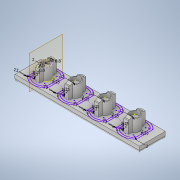
# Autodesk Inventor part: CapsFor24WellPlate
Saved by Autodesk Inventor 2021 (Build 250183000, 183)
## iProperties
Created: 2019-12-10
Part Number: CapsFor24WellPlate
Material: Generic
Document SubType Name: Modeling
Designer: Sergio
Density: 1 g/cm^3
Appearance: Default
Author: Sergio
Autodesk Inventor part; units mm, degrees
ref_plane "YZ Plane" through (0, 0, 0) normal (1, 0, 0) x (0, 1, 0)
ref_plane "XZ Plane" through (0, 0, 0) normal (0, 1, 0) x (-1, 0, 0)
ref_plane "XY Plane" through (0, 0, 0) normal (0, 0, 1) x (1, 0, 0)
sketch "Sketch1" plane through (0, 0, 0) normal (0, 1, 0) x (-1, 0, 0)
  circle A0 centre (-29.25, 0) radius 2.8 construction
  circle A1 centre (-9.75, 0) radius 2.8 construction
  circle A2 centre (9.75, 0) radius 2.8 construction
  circle A3 centre (29.25, 0) radius 2.8 construction
  line L0 (-29.25, 0) -> (29.25, 0) construction
  line L1 (29.25, 0) -> (29.25, -4.8) construction
  line L2 (9.75, 0) -> (9.75, -4.8) construction
  line L3 (-9.75, 0) -> (-9.75, -4.8) construction
  line L4 (-29.25, 0) -> (-29.25, -4.8) construction
  line L5 (29.25, 0) -> (29.25, 4.8) construction
  line L6 (9.75, 0) -> (9.75, 4.8) construction
  line L7 (-9.75, 0) -> (-9.75, 4.8) construction
  line L8 (-29.25, 0) -> (-29.25, 4.8) construction
  line L9 (30.65, -5.6) -> (27.85, -5.6) construction
  line L10 (27.85, -5.6) -> (27.85, -4.8) construction
  line L11 (27.85, -4.8) -> (30.65, -4.8) construction
  line L12 (30.65, -4.8) -> (30.65, -5.6) construction
  line L13 (11.15, -5.6) -> (8.35, -5.6) construction
  line L14 (8.35, -5.6) -> (8.35, -4.8) construction
  line L15 (8.35, -4.8) -> (11.15, -4.8) construction
  line L16 (11.15, -4.8) -> (11.15, -5.6) construction
  line L17 (-8.35, -5.6) -> (-11.15, -5.6) construction
  line L18 (-11.15, -5.6) -> (-11.15, -4.8) construction
  line L19 (-11.15, -4.8) -> (-8.35, -4.8) construction
  line L20 (-8.35, -4.8) -> (-8.35, -5.6) construction
  line L21 (-27.85, -5.6) -> (-30.65, -5.6) construction
  line L22 (-30.65, -5.6) -> (-30.65, -4.8) construction
  line L23 (-30.65, -4.8) -> (-27.85, -4.8) construction
  line L24 (-27.85, -4.8) -> (-27.85, -5.6) construction
  line L25 (27.85, 5.6) -> (30.65, 5.6) construction
  line L26 (30.65, 5.6) -> (30.65, 4.8) construction
  line L27 (30.65, 4.8) -> (27.85, 4.8) construction
  line L28 (27.85, 4.8) -> (27.85, 5.6) construction
  line L29 (8.35, 5.6) -> (11.15, 5.6) construction
  line L30 (11.15, 5.6) -> (11.15, 4.8) construction
  line L31 (11.15, 4.8) -> (8.35, 4.8) construction
  line L32 (8.35, 4.8) -> (8.35, 5.6) construction
  line L33 (-11.15, 5.6) -> (-8.35, 5.6) construction
  line L34 (-8.35, 5.6) -> (-8.35, 4.8) construction
  line L35 (-8.35, 4.8) -> (-11.15, 4.8) construction
  line L36 (-11.15, 4.8) -> (-11.15, 5.6) construction
  line L37 (-30.65, 5.6) -> (-27.85, 5.6) construction
  line L38 (-27.85, 5.6) -> (-27.85, 4.8) construction
  line L39 (-27.85, 4.8) -> (-30.65, 4.8) construction
  line L40 (-30.65, 4.8) -> (-30.65, 5.6) construction
  dimension "d171" = 2.8
  dimension "d172" = 0.8
  dimension "d173" = 2.8
  dimension "d174" = 0.8
  dimension "d175" = 2.8
  dimension "d176" = 0.8
  dimension "d177" = 2.8
  dimension "d178" = 0.8
  dimension "d179" = 2.8
  dimension "d180" = 0.8
  dimension "d181" = 2.8
  dimension "d182" = 0.8
  dimension "d183" = 2.8
  dimension "d184" = 0.8
  dimension "d185" = 2.8
  dimension "d186" = 0.8
  constraints: 82 end point, 16 parallel, 8 midpoint, 8 perpendicular, 5 horizontal, 4 centre point, 4 vertical
  measures "d171" distance of L10.end L11.end
  measures "d172" distance of L10.start L10.end
  measures "d173" distance of L14.end L15.end
  measures "d174" distance of L14.start L14.end
  measures "d175" distance of L18.end L19.end
  measures "d176" distance of L18.start L18.end
  measures "d177" distance of L22.end L23.end
  measures "d178" distance of L22.start L22.end
  measures "d179" distance of L27.start L28.start
  measures "d180" distance of L25.end L27.start
  measures "d181" distance of L31.start L32.start
  measures "d182" distance of L29.end L31.start
  measures "d183" distance of L35.start L36.start
  measures "d184" distance of L33.end L35.start
  measures "d185" distance of L39.start L40.start
  measures "d186" distance of L37.end L39.start
sketch "Sketch26" plane through (0, 0, 0) normal (0, 1, 0) x (-1, 0, 0)
  line L0 (-41, -8.5) -> (41, -8.5)
  line L1 (41, -8.5) -> (41, 8.5)
  line L2 (41, 8.5) -> (-41, 8.5)
  line L3 (-41, 8.5) -> (-41, -8.5)
  line L4 (-41, -8.5) -> (41, 8.5) construction
  line L5 (41, -8.5) -> (-41, 8.5) construction
  point P0 (0, 0)
  dimension "d187" = 82
  dimension "d188" = 17
  constraints: 12 end point, 2 midpoint, 2 parallel, 1 horizontal, 1 perpendicular
  measures "d187" distance of L2.end L1.end
  measures "d188" distance of L1.end L0.end
extrude "Extrusion11" add sketch "Sketch26" against normal blind 4.5
sketch "Sketch27" plane through (0, 0, 0) normal (0, 1, 0) x (1, 0, 0)
  circle A0 centre (-29.25, 0) radius 2.8 construction
  circle A1 centre (-9.75, 0) radius 2.8 construction
  circle A2 centre (9.75, 0) radius 2.8 construction
  circle A3 centre (29.25, 0) radius 2.8 construction
  line L0 (-30.65, 5.6) -> (-27.85, 5.6) construction
  line L1 (-27.85, 4.8) -> (-30.65, 4.8) construction
  line L2 (-11.15, 5.6) -> (-8.35, 5.6) construction
  line L3 (-8.35, 4.8) -> (-11.15, 4.8) construction
  line L4 (8.35, 5.6) -> (11.15, 5.6) construction
  line L5 (11.15, 4.8) -> (8.35, 4.8) construction
  line L6 (30.65, 4.8) -> (27.85, 4.8) construction
  line L7 (27.85, 5.6) -> (30.65, 5.6) construction
  line L8 (-27.85, -5.6) -> (-30.65, -5.6) construction
  line L9 (-30.65, -4.8) -> (-27.85, -4.8) construction
  circle A4 centre (-29.25, 0) radius 3.325
  circle A5 centre (-9.75, 0) radius 3.325
  circle A6 centre (9.75, 0) radius 3.325
  circle A7 centre (29.25, 0) radius 3.325
  line L10 (-11.15, 5.6) -> (-8.35, 5.6)
  line L11 (-8.35, 5.6) -> (-8.35, 4.8)
  line L12 (-8.35, 4.8) -> (-11.15, 4.8)
  line L13 (-11.15, 4.8) -> (-11.15, 5.6)
  line L14 (8.35, 5.6) -> (11.15, 5.6)
  line L15 (11.15, 5.6) -> (11.15, 4.8)
  line L16 (11.15, 4.8) -> (8.35, 4.8)
  line L17 (8.35, 4.8) -> (8.35, 5.6)
  line L18 (27.85, 5.6) -> (30.65, 5.6)
  line L19 (30.65, 5.6) -> (30.65, 4.8)
  line L20 (30.65, 4.8) -> (27.85, 4.8)
  line L21 (27.85, 4.8) -> (27.85, 5.6)
  line L22 (-30.65, 5.6) -> (-27.85, 5.6)
  line L23 (-27.85, 5.6) -> (-27.85, 4.8)
  line L24 (-27.85, 4.8) -> (-30.65, 4.8)
  line L25 (-30.65, 4.8) -> (-30.65, 5.6)
  line L26 (-30.65, -4.8) -> (-27.85, -4.8)
  line L27 (-27.85, -4.8) -> (-27.85, -5.6)
  line L28 (-27.85, -5.6) -> (-30.65, -5.6)
  line L29 (-30.65, -5.6) -> (-30.65, -4.8)
  line L30 (-8.35, -5.6) -> (-11.15, -5.6) construction
  line L31 (-11.15, -4.8) -> (-8.35, -4.8) construction
  line L32 (11.15, -5.6) -> (8.35, -5.6) construction
  line L33 (8.35, -4.8) -> (11.15, -4.8) construction
  line L34 (30.65, -5.6) -> (27.85, -5.6) construction
  line L35 (27.85, -4.8) -> (30.65, -4.8) construction
  line L36 (-11.15, -4.8) -> (-8.35, -4.8)
  line L37 (-8.35, -4.8) -> (-8.35, -5.6)
  line L38 (-8.35, -5.6) -> (-11.15, -5.6)
  line L39 (-11.15, -5.6) -> (-11.15, -4.8)
  line L40 (8.35, -4.8) -> (11.15, -4.8)
  line L41 (11.15, -4.8) -> (11.15, -5.6)
  line L42 (11.15, -5.6) -> (8.35, -5.6)
  line L43 (8.35, -5.6) -> (8.35, -4.8)
  line L44 (27.85, -4.8) -> (30.65, -4.8)
  line L45 (30.65, -4.8) -> (30.65, -5.6)
  line L46 (30.65, -5.6) -> (27.85, -5.6)
  line L47 (27.85, -5.6) -> (27.85, -4.8)
  line L48 (-30.65, 4.8) -> (-30.65, -4.8)
  line L49 (-27.85, 4.8) -> (-27.85, -4.8)
  line L50 (-11.15, 4.8) -> (-11.15, -4.8)
  line L51 (-8.35, 4.8) -> (-8.35, -4.8)
  line L52 (27.85, 4.8) -> (27.85, -4.8)
  line L53 (30.65, -4.8) -> (30.65, 4.8)
  line L54 (8.35, 4.8) -> (8.35, -4.8)
  line L55 (11.15, -4.8) -> (11.15, 4.8)
  point P0 (0, 0)
  dimension "d191" = 6.65
  dimension "d192" = 6.65
  dimension "d193" = 6.65
  dimension "d194" = 6.65
  constraints: 80 end point, 22 parallel, 10 perpendicular, 8 horizontal, 4 centre point, 4 coincident
  measures "d191" diameter of A4
  measures "d192" diameter of A5
  measures "d193" diameter of A6
  measures "d194" diameter of A7
extrude "Extrusion12" add sketch "Sketch27" along normal blind 8
sketch "Sketch28" plane through (0, 8, 0) normal (0, 1, 0) x (1, 0, 0)
  arc A0 (-30.65, 3.0159) -> (-30.65, -3.0159) centre (-29.25, 0) ccw projected
  circle A1 centre (-29.25, 0) radius 2.825
  arc A2 (-8.35, -3.0159) -> (-8.35, 3.0159) centre (-9.75, 0) ccw projected
  circle A3 centre (-9.75, 0) radius 2.825
  arc A4 (11.15, -3.0159) -> (11.15, 3.0159) centre (9.75, 0) ccw projected
  circle A5 centre (9.75, 0) radius 2.825
  arc A6 (30.65, -3.0159) -> (30.65, 3.0159) centre (29.25, 0) ccw projected
  circle A7 centre (29.25, 0) radius 2.825
  point P0 (0, 0)
  dimension "d197" = 5.65
  dimension "d198" = 5.65
  dimension "d199" = 5.65
  dimension "d200" = 5.65
  constraints: 4 centre point, 4 coincident
  measures "d197" diameter of A1
  measures "d198" diameter of A3
  measures "d199" diameter of A5
  measures "d200" diameter of A7
extrude "Extrusion13" cut sketch "Sketch28" against normal blind 2
sketch "Sketch29" plane through (0, 8, 0) normal (0, 1, 0) x (1, 0, 0)
  line L0 (-27.85, 5.6) -> (-30.65, 5.6) construction
  line L1 (-30.65, 5.6) -> (-27.85, 5.6) construction
  line L2 (-27.85, 5.6) -> (-27.85, 4.8) construction
  line L3 (-27.85, 4.8) -> (-30.65, 4.8) construction
  line L4 (-30.65, 4.8) -> (-30.65, 5.6) construction
  line L5 (-30.65, -3.0159) -> (-30.65, -5.6) construction
  line L6 (-30.65, -5.6) -> (-27.85, -5.6) construction
  line L7 (-27.85, -5.6) -> (-27.85, -4.8) construction
  line L8 (-27.85, -4.8) -> (-30.65, -4.8) construction
  line L9 (-30.65, -4.8) -> (-30.65, -5.6) construction
  arc A0 (-27.85, -3.0159) -> (-27.85, 3.0159) centre (-29.25, 0) ccw construction
  circle A1 centre (-29.25, 0) radius 3.325 construction
  line L10 (-29.25, 0) -> (-26.425, 0) construction
  circle A2 centre (-29.25, 0) radius 2.825 construction
  point P0 (-9.75, 0)
  point P1 (9.75, 0)
  point P2 (29.25, 0)
  dimension "d203" = 2.8
  dimension "d204" = 0.8
  dimension "d205" = 2.8
  dimension "d206" = 0.8
  constraints: 18 end point, 4 parallel, 3 horizontal, 2 coincident, 2 perpendicular, 1 centre point, 1 horizontal alignment, 1 other
  measures "d203" distance of L2.end L3.end
  measures "d204" distance of L1.end L2.end
  measures "d205" distance of L8.end L7.end
  measures "d206" distance of L7.end L6.end
ref_plane "Work Plane7" through (-29.25, 8, 0) normal (1, 0, 0) x (0, 1, 0)
sketch "Sketch30" plane through (-29.25, 8, 0) normal (1, 0, 0) x (0, 1, 0)
  line L0 (0, -3.325) -> (0, 3.325) construction
  line L1 (0, 4.8) -> (0, 3.325)
  line L2 (0, 3.325) -> (1, 3.325)
  line L3 (1, 3.325) -> (0, 4.8)
  line L4 (0, -4.8) -> (0, -3.325)
  line L5 (0, -3.325) -> (1, -3.325)
  line L6 (1, -3.325) -> (0, -4.8)
  point P0 (-8, 0)
  dimension "d207" = 1
  dimension "d210" = 1
  constraints: 12 end point, 2 vertical, 1 horizontal, 1 perpendicular
  measures "d207" distance of L0.end L2.end
  measures "d210" distance of L0.start L5.end
extrude "Extrusion14" add sketch "Sketch30" along normal mid plane 2.8 contours L3 L2 L1
extrude "Extrusion15" add sketch "Sketch30" along normal mid plane 2.8 contours L4 L5 L6
sketch "Sketch31" plane through (0, 8, 0) normal (0, 1, 0) x (1, 0, 0)
  line L0 (-30.65, -3.325) -> (-27.85, -3.325) projected
  arc A0 (-27.85, -3.0159) -> (-27.85, 3.0159) centre (-29.25, 0) ccw projected
  line L1 (-27.85, -3.325) -> (-27.85, -3.0159) projected
  line L2 (-27.85, -3.325) -> (-27.85, -3.0159)
  line L3 (-27.85, -3.325) -> (-29.25, -3.325)
  line L4 (-30.65, -3.0159) -> (-30.65, -3.325) projected
  arc A1 (-30.65, 3.0159) -> (-30.65, -3.0159) centre (-29.25, 0) ccw projected
  line L5 (-30.65, -3.0159) -> (-30.65, -3.325)
  line L6 (-30.65, -3.325) -> (-29.25, -3.325)
  line L7 (-27.85, 3.325) -> (-30.65, 3.325) projected
  line L8 (-30.65, 3.0159) -> (-30.65, 3.325)
  line L9 (-27.85, 3.0159) -> (-27.85, 3.325)
  line L10 (-27.85, 3.325) -> (-29.25, 3.325)
  line L11 (-29.25, 3.325) -> (-30.65, 3.325)
  line L12 (-30.65, -3.0159) -> (-30.65, -2.4537)
  circle A2 centre (-29.25, 0) radius 2.825 projected
  line L13 (-27.85, -3.0159) -> (-27.85, -2.4537)
  arc A3 (-30.65, -2.4537) -> (-27.85, -2.4537) centre (-29.25, 0) ccw
  line L14 (-30.65, 3.0159) -> (-30.65, 2.4537)
  line L15 (-27.85, 3.0159) -> (-27.85, 2.4537)
  arc A4 (-27.85, 2.4537) -> (-30.65, 2.4537) centre (-29.25, 0) ccw
  point P0 (0, 0)
  constraints: 24 end point, 8 point on circle, 3 collinear, 3 perpendicular, 3 vertical, 2 centre point, 2 concentric, 2 midpoint, 1 parallel, 1 point on line
fillet "Fillet2" radius 2 4 edges at (0, -4.5, -8.5) (0, -4.5, 8.5) (41, -4.5, 0) (-41, -4.5, 0)
sketch "Sketch33" plane through (0, 8, 0) normal (0, 1, 0) x (1, 0, 0)
  circle A0 centre (-9.75, 0) radius 2.825 projected
  circle A1 centre (9.75, 0) radius 2.825 projected
  circle A2 centre (29.25, 0) radius 2.825 projected
  point P0 (0, 0)
  constraints: 3 coincident
extrude "Extrusion19" add sketch "Sketch31" along normal blind 1 contours L4 L12 A2 L13 L1 L0 | L8 L7 L9 L15 A2 L14
pattern_sketch "Sketch Driven Pattern3" of "Extrusion14", "Extrusion19", "Extrusion15" from (-29.25, 8, 0) copies at (-9.75, 8, 0) at (9.75, 8, 0) at (29.25, 8, 0)
sketch "Sketch34" plane through (0, 0, 0) normal (0, 1, 0) x (1, 0, 0)
  circle A0 centre (-29.25, 0) radius 2.8 construction
  line L0 (-22, 0) -> (-26.45, 0) construction
  arc A1 (-30.65, 3.0159) -> (-30.65, -3.0159) centre (-29.25, 0) ccw projected
  line L1 (-32.575, 0) -> (-34.575, 0) construction
  line L2 (-34.575, 0) -> (-34.575, 4.0629)
  line L3 (-34.575, 0) -> (-34.575, -4.0629)
  line L4 (-34.575, 0) -> (-35.825, 0) construction
  line L5 (-35.825, 0) -> (-35.825, 4.6173)
  line L6 (-35.825, 0) -> (-35.825, -4.6173)
  arc A2 (-35.825, -4.6173) -> (-35.2327, -6.038) centre (-33.825, -4.6173) ccw
  arc A3 (-34.575, -4.0629) -> (-33.8417, -5.6106) centre (-32.575, -4.0629) ccw
  arc A4 (-33.8417, 5.6106) -> (-34.575, 4.0629) centre (-32.575, 4.0629) ccw
  arc A5 (-35.2327, 6.038) -> (-35.825, 4.6173) centre (-33.825, 4.6173) ccw
  arc A6 (-27.85, -3.0159) -> (-27.85, 3.0159) centre (-29.25, 0) ccw projected
  line L7 (-25.925, 0) -> (-23.925, 0) construction
  line L8 (-23.925, 0) -> (-22.675, 0) construction
  line L9 (-23.925, 0) -> (-23.925, 4.0629)
  line L10 (-23.925, 0) -> (-23.925, -4.0629)
  line L11 (-22.675, 0) -> (-22.675, 4.6173)
  line L12 (-22.675, 0) -> (-22.675, -4.6173)
  arc A7 (-35.2327, -6.038) -> (-23.2673, -6.038) centre (-29.25, 0) ccw
  arc A8 (-23.2673, 6.038) -> (-35.2327, 6.038) centre (-29.25, 0) ccw
  arc A9 (-33.8417, -5.6106) -> (-24.6583, -5.6106) centre (-29.25, 0) ccw
  arc A10 (-24.6583, 5.6106) -> (-33.8417, 5.6106) centre (-29.25, 0) ccw
  arc A11 (-24.6583, -5.6106) -> (-23.925, -4.0629) centre (-25.925, -4.0629) ccw
  arc A12 (-23.2673, -6.038) -> (-22.675, -4.6173) centre (-24.675, -4.6173) ccw
  arc A13 (-22.675, 4.6173) -> (-23.2673, 6.038) centre (-24.675, 4.6173) ccw
  arc A14 (-23.925, 4.0629) -> (-24.6583, 5.6106) centre (-25.925, 4.0629) ccw
  circle A15 centre (-32.575, -4.0629) radius 1
  circle A16 centre (-9.75, 0) radius 2.825 projected
  circle A17 centre (9.75, 0) radius 2.825 projected
  circle A18 centre (29.25, 0) radius 2.825 projected
  line L13 (-2.5, 0) -> (-6.95, 0) construction
  line L14 (-13.075, 0) -> (-15.075, 0) construction
  line L15 (-15.075, 0) -> (-15.075, 4.0629)
  line L16 (-15.075, 0) -> (-15.075, -4.0629)
  line L17 (-15.075, 0) -> (-16.325, 0) construction
  line L18 (-16.325, 0) -> (-16.325, 4.6173)
  line L19 (-16.325, 0) -> (-16.325, -4.6173)
  arc A19 (-16.325, -4.6173) -> (-15.7327, -6.038) centre (-14.325, -4.6173) ccw
  arc A20 (-15.075, -4.0629) -> (-14.3417, -5.6106) centre (-13.075, -4.0629) ccw
  arc A21 (-14.3417, 5.6106) -> (-15.075, 4.0629) centre (-13.075, 4.0629) ccw
  arc A22 (-15.7327, 6.038) -> (-16.325, 4.6173) centre (-14.325, 4.6173) ccw
  line L20 (-6.425, 0) -> (-4.425, 0) construction
  line L21 (-4.425, 0) -> (-3.175, 0) construction
  line L22 (-4.425, 0) -> (-4.425, 4.0629)
  line L23 (-4.425, 0) -> (-4.425, -4.0629)
  line L24 (-3.175, 0) -> (-3.175, 4.6173)
  line L25 (-3.175, 0) -> (-3.175, -4.6173)
  arc A23 (-15.7327, -6.038) -> (-3.7673, -6.038) centre (-9.75, 0) ccw
  arc A24 (-3.7673, 6.038) -> (-15.7327, 6.038) centre (-9.75, 0) ccw
  arc A25 (-14.3417, -5.6106) -> (-5.1583, -5.6106) centre (-9.75, 0) ccw
  arc A26 (-5.1583, 5.6106) -> (-14.3417, 5.6106) centre (-9.75, 0) ccw
  arc A27 (-5.1583, -5.6106) -> (-4.425, -4.0629) centre (-6.425, -4.0629) ccw
  arc A28 (-3.7673, -6.038) -> (-3.175, -4.6173) centre (-5.175, -4.6173) ccw
  arc A29 (-3.175, 4.6173) -> (-3.7673, 6.038) centre (-5.175, 4.6173) ccw
  arc A30 (-4.425, 4.0629) -> (-5.1583, 5.6106) centre (-6.425, 4.0629) ccw
  circle A31 centre (-13.075, -4.0629) radius 1
  line L26 (17, 0) -> (12.55, 0) construction
  line L27 (6.425, 0) -> (4.425, 0) construction
  line L28 (4.425, 0) -> (4.425, 4.0629)
  line L29 (4.425, 0) -> (4.425, -4.0629)
  line L30 (4.425, 0) -> (3.175, 0) construction
  line L31 (3.175, 0) -> (3.175, 4.6173)
  line L32 (3.175, 0) -> (3.175, -4.6173)
  arc A32 (3.175, -4.6173) -> (3.7673, -6.038) centre (5.175, -4.6173) ccw
  arc A33 (4.425, -4.0629) -> (5.1583, -5.6106) centre (6.425, -4.0629) ccw
  arc A34 (5.1583, 5.6106) -> (4.425, 4.0629) centre (6.425, 4.0629) ccw
  arc A35 (3.7673, 6.038) -> (3.175, 4.6173) centre (5.175, 4.6173) ccw
  line L33 (13.075, 0) -> (15.075, 0) construction
  line L34 (15.075, 0) -> (16.325, 0) construction
  line L35 (15.075, 0) -> (15.075, 4.0629)
  line L36 (15.075, 0) -> (15.075, -4.0629)
  line L37 (16.325, 0) -> (16.325, 4.6173)
  line L38 (16.325, 0) -> (16.325, -4.6173)
  arc A36 (3.7673, -6.038) -> (15.7327, -6.038) centre (9.75, 0) ccw
  arc A37 (15.7327, 6.038) -> (3.7673, 6.038) centre (9.75, 0) ccw
  arc A38 (5.1583, -5.6106) -> (14.3417, -5.6106) centre (9.75, 0) ccw
  arc A39 (14.3417, 5.6106) -> (5.1583, 5.6106) centre (9.75, 0) ccw
  arc A40 (14.3417, -5.6106) -> (15.075, -4.0629) centre (13.075, -4.0629) ccw
  arc A41 (15.7327, -6.038) -> (16.325, -4.6173) centre (14.325, -4.6173) ccw
  arc A42 (16.325, 4.6173) -> (15.7327, 6.038) centre (14.325, 4.6173) ccw
  arc A43 (15.075, 4.0629) -> (14.3417, 5.6106) centre (13.075, 4.0629) ccw
  circle A44 centre (6.425, -4.0629) radius 1
  line L39 (36.5, 0) -> (32.05, 0) construction
  line L40 (25.925, 0) -> (23.925, 0) construction
  line L41 (23.925, 0) -> (23.925, 4.0629)
  line L42 (23.925, 0) -> (23.925, -4.0629)
  line L43 (23.925, 0) -> (22.675, 0) construction
  line L44 (22.675, 0) -> (22.675, 4.6173)
  line L45 (22.675, 0) -> (22.675, -4.6173)
  arc A45 (22.675, -4.6173) -> (23.2673, -6.038) centre (24.675, -4.6173) ccw
  arc A46 (23.925, -4.0629) -> (24.6583, -5.6106) centre (25.925, -4.0629) ccw
  arc A47 (24.6583, 5.6106) -> (23.925, 4.0629) centre (25.925, 4.0629) ccw
  arc A48 (23.2673, 6.038) -> (22.675, 4.6173) centre (24.675, 4.6173) ccw
  line L46 (32.575, 0) -> (34.575, 0) construction
  line L47 (34.575, 0) -> (35.825, 0) construction
  line L48 (34.575, 0) -> (34.575, 4.0629)
  line L49 (34.575, 0) -> (34.575, -4.0629)
  line L50 (35.825, 0) -> (35.825, 4.6173)
  line L51 (35.825, 0) -> (35.825, -4.6173)
  arc A49 (23.2673, -6.038) -> (35.2327, -6.038) centre (29.25, 0) ccw
  arc A50 (35.2327, 6.038) -> (23.2673, 6.038) centre (29.25, 0) ccw
  arc A51 (24.6583, -5.6106) -> (33.8417, -5.6106) centre (29.25, 0) ccw
  arc A52 (33.8417, 5.6106) -> (24.6583, 5.6106) centre (29.25, 0) ccw
  arc A53 (33.8417, -5.6106) -> (34.575, -4.0629) centre (32.575, -4.0629) ccw
  arc A54 (35.2327, -6.038) -> (35.825, -4.6173) centre (33.825, -4.6173) ccw
  arc A55 (35.825, 4.6173) -> (35.2327, 6.038) centre (33.825, 4.6173) ccw
  arc A56 (34.575, 4.0629) -> (33.8417, 5.6106) centre (32.575, 4.0629) ccw
  circle A57 centre (25.925, -4.0629) radius 1
  point P0 (-35.825, 5.387)
  point P1 (-35.825, -5.387)
  point P2 (-34.575, 4.92)
  point P3 (-34.575, -4.92)
  point P4 (-22.675, 5.387)
  point P5 (-22.675, -5.387)
  point P6 (-23.925, 4.92)
  point P7 (-23.925, -4.92)
  point P8 (-16.325, 5.387)
  point P9 (-16.325, -5.387)
  point P10 (-15.075, 4.92)
  point P11 (-15.075, -4.92)
  point P12 (-3.175, 5.387)
  point P13 (-3.175, -5.387)
  point P14 (-4.425, 4.92)
  point P15 (-4.425, -4.92)
  point P16 (3.175, 5.387)
  point P17 (3.175, -5.387)
  point P18 (4.425, 4.92)
  point P19 (4.425, -4.92)
  point P20 (16.325, 5.387)
  point P21 (16.325, -5.387)
  point P22 (15.075, 4.92)
  point P23 (15.075, -4.92)
  point P24 (22.675, 5.387)
  point P25 (22.675, -5.387)
  point P26 (23.925, 4.92)
  point P27 (23.925, -4.92)
  point P28 (35.825, 5.387)
  point P29 (35.825, -5.387)
  point P30 (34.575, 4.92)
  point P31 (34.575, -4.92)
  dimension "d242" = 2
  dimension "d243" = 1.25
  dimension "d244" = 2
  dimension "d245" = 2
  dimension "d246" = 2
  dimension "d247" = 2
  dimension "d248" = 1.25
  dimension "d249" = 2
  dimension "d250" = 2
  dimension "d251" = 2
  dimension "d252" = 1.25
  dimension "d253" = 2
  dimension "d254" = 2
  dimension "d255" = 2
  dimension "d256" = 2
  dimension "d257" = 1.25
  dimension "d258" = 2
  dimension "d259" = 2
  dimension "d260" = 2
  dimension "d261" = 1.25
  dimension "d262" = 2
  dimension "d263" = 2
  dimension "d264" = 2
  dimension "d265" = 2
  dimension "d266" = 1.25
  dimension "d267" = 2
  dimension "d268" = 2
  dimension "d269" = 2
  dimension "d270" = 1.25
  dimension "d271" = 2
  dimension "d272" = 2
  dimension "d273" = 2
  dimension "d274" = 2
  dimension "d275" = 1.25
  dimension "d276" = 2
  dimension "d277" = 2
  constraints: 114 point on circle, 104 end point, 52 centre point, 48 point on line, 48 tangent, 24 vertical, 16 equal radius, 12 coincident, 8 horizontal, 1 horizontal alignment, 1 other
  measures "d242" distance of L1.start L1.end
  measures "d243" distance of L1.end L4.end
  measures "d244" radius of A2
  measures "d245" radius of A3
  measures "d246" radius of A4
  measures "d247" distance of L7.start L7.end
  measures "d248" distance of L7.end L8.end
  measures "d249" radius of A11
  measures "d250" diameter of A15
  measures "d251" distance of L14.start L14.end
  measures "d252" distance of L14.end L17.end
  measures "d253" radius of A19
  measures "d254" radius of A20
  measures "d255" radius of A21
  measures "d256" distance of L20.start L20.end
  measures "d257" distance of L20.end L24.start
  measures "d258" radius of A27
  measures "d259" diameter of A31
  measures "d260" distance of L27.start L27.end
  measures "d261" distance of L27.end L30.end
  measures "d262" radius of A32
  measures "d263" radius of A33
  measures "d264" radius of A34
  measures "d265" distance of L33.start L33.end
  measures "d266" distance of L33.end L37.start
  measures "d267" radius of A40
  measures "d268" diameter of A44
  measures "d269" distance of L40.start L40.end
  measures "d270" distance of L40.end L43.end
  measures "d271" radius of A45
  measures "d272" radius of A46
  measures "d273" radius of A47
  measures "d274" distance of L46.start L46.end
  measures "d275" distance of L46.end L50.start
  measures "d276" radius of A53
  measures "d277" diameter of A57
body "Solid4"
